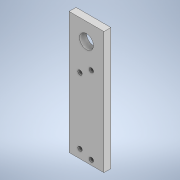
# Autodesk Inventor part: DoorMotorDriveCase
Saved by Autodesk Inventor 2020 (Build 240168000, 168)
## iProperties
Created: 2019-10-16
Part Number: DoorMotorDriveCase
Material: 일반
Document SubType Name: Modeling
Designer: Knowblesse
Density: 1 g/cm^3
Appearance: 기본값
Author: Knowblesse
## iProperties of the stored document _3D 인쇄.ipt
Created: 2019-10-16
Part Number: _3D 인쇄
Material: 일반
Document SubType Name: Modeling
Designer: Knowblesse
Density: 1 g/cm^3
Appearance: 기본값
Author: Knowblesse
Autodesk Inventor part; units mm, degrees
ref_plane "YZ Plane" through (0, 0, 0) normal (1, 0, 0) x (0, 1, 0)
ref_plane "XZ Plane" through (0, 0, 0) normal (0, 1, 0) x (-1, 0, 0)
ref_plane "XY Plane" through (0, 0, 0) normal (0, 0, 1) x (1, 0, 0)
sketch "스케치1" plane through (0, 0, 0) normal (0, 0, 1) x (1, 0, 0)
  line L0 (0, 0) -> (20, 0)
  line L1 (20, 0) -> (20, 50)
  line L2 (20, 50) -> (0, 50)
  line L3 (0, 50) -> (0, 0)
  dimension "d0" = 20
  dimension "d1" = 50
  constraints: 8 end point, 2 parallel, 1 horizontal, 1 perpendicular
  measures "d0" distance of L2.end L1.end
  measures "d1" distance of L1.end L0.end
extrude "돌출1" add sketch "스케치1" along normal blind 4
sketch "스케치2" plane through (0, 0, 4) normal (0, 0, 1) x (1, 0, 0)
  line L0 (0, 0) -> (20, 0) projected
  line L1 (20, 0) -> (20, 50) projected
  line L2 (20, 50) -> (0, 50) projected
  line L3 (0, 50) -> (0, 0) projected
  line L4 (20, 50) -> (0, 50) construction
  line L5 (10, 50) -> (10, 0) construction
  point P0 (6.3, 42.8)
  point P1 (6.3, 5)
  point P2 (12.8, 47.2)
  point P3 (12.8, 2.8)
  dimension "d4" = 2.8
  dimension "d5" = 2.8
  dimension "d6" = 2.8
  dimension "d7" = 5
  dimension "d8" = 7.2
  dimension "d9" = 3.7
  constraints: 2 end point, 2 midpoint, 2 vertical alignment
  measures "d4" distance from line of point (12.8, 2.8) L0
  measures "d5" distance from line of L2 point (12.8, 47.2)
  measures "d6" distance from line of L5 point (12.8, 47.2)
  measures "d7" distance from line of point (6.3, 5) L0
  measures "d8" distance from line of L2 point (6.3, 42.8)
  measures "d9" distance from line of L5 point (6.3, 42.8)
hole "구멍1" at (6.3, 42.8, 4) at (6.3, 5, 4) at (12.8, 47.2, 4) at (12.8, 2.8, 4) direction (0, 0, -1) diameter 2.5 end through all
sketch "스케치3" plane through (0, 50, 0) normal (0, 1, 0) x (1, 0, 0)
  line L0 (20, 0) -> (0, 0) projected
  line L1 (0, 0) -> (0, -4) projected
  line L2 (20, -4) -> (0, -4) projected
  line L3 (20, 0) -> (20, -4) projected
extrude "돌출2" add sketch "스케치3" along normal blind 20
sketch "스케치4" plane through (0, 0, 4) normal (0, 0, 1) x (1, 0, 0)
  line L0 (0, 70) -> (20, 70) projected
  point P0 (0, 0)
  point P1 (10, 60)
  point P2 (10, 70)
  dimension "d19" = 10
  constraints: 1 midpoint, 1 vertical alignment
  measures "d19" distance from line of L0 point (10, 60)
hole "구멍2" at (10, 60, 4) direction (0, 0, -1) diameter 8 end through all
